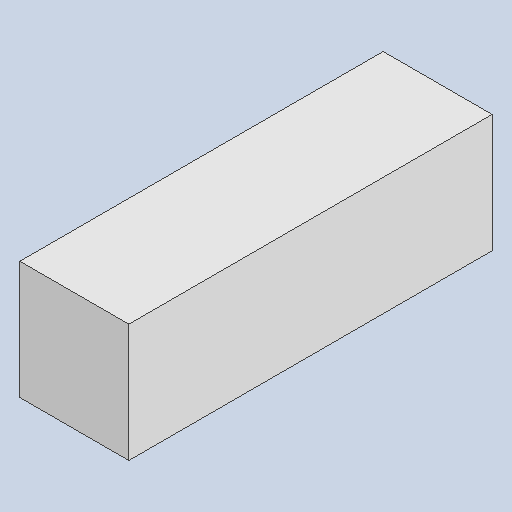
# Autodesk Inventor part: lipol 150mAH
Saved by Autodesk Inventor 2023 (Build 270158000, 158)
## iProperties
Created: 2022-12-13
Part Number: lipol 150mAH
Material: Generic
Document SubType Name: Modeling
Designer: komputer
Density: 1 g/cm^3
Appearance: Default
Author: komputer
Autodesk Inventor part; units mm, degrees
ref_plane "YZ Plane" through (0, 0, 0) normal (1, 0, 0) x (0, 1, 0)
ref_plane "XZ Plane" through (0, 0, 0) normal (0, 1, 0) x (-1, 0, 0)
ref_plane "XY Plane" through (0, 0, 0) normal (0, 0, 1) x (1, 0, 0)
sketch "Sketch1" plane through (0, 0, 0) normal (0, 0, 1) x (1, 0, 0)
  line L0 (-2.9135, 2.0782) -> (9.0865, 2.0782)
  line L1 (9.0865, 2.0782) -> (9.0865, -10.9218)
  line L2 (9.0865, -10.9218) -> (-2.9135, -10.9218)
  line L3 (-2.9135, -10.9218) -> (-2.9135, 2.0782)
  point P0 (0, 0)
  dimension "d0" = 12
  dimension "d1" = 13
  constraints: 8 end point, 2 parallel, 1 horizontal, 1 perpendicular
  measures "d0" distance of L1.end L2.end
  measures "d1" distance of L0.end L1.end
extrude "Extrusion1" add sketch "Sketch1" along normal blind 40
body "Solid1"
